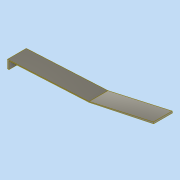
# Autodesk Inventor part: limitSwitchTrigger
Saved by Autodesk Inventor 2017 (Build 210142000, 142)
## iProperties
Created: 2016-12-03
Part Number: limitSwitchTrigger
Material: Steel
Document SubType Name: Modeling
Designer: techn
Density: 7.85 g/cm^3
Appearance: Silver
Author: techn
Autodesk Inventor part; units mm, degrees
ref_plane "YZ Plane" through (0, 0, 0) normal (1, 0, 0) x (0, 1, 0)
ref_plane "XZ Plane" through (0, 0, 0) normal (0, 1, 0) x (-1, 0, 0)
ref_plane "XY Plane" through (0, 0, 0) normal (0, 0, 1) x (1, 0, 0)
sketch "Sketch1" plane through (0, 0, 0) normal (0, 0, 1) x (1, 0, 0)
  line L0 (0, 0) -> (0, 1.016)
  line L1 (0, 1.016) -> (10.8309, 1.5836)
  line L2 (10.8309, 1.5836) -> (19.5267, 3.432)
  line L3 (10.8309, 1.5836) -> (19.7209, 1.5836) construction
  line L4 (19.5267, 3.432) -> (19.4844, 3.6307)
  line L5 (19.4844, 3.6307) -> (10.8098, 1.683)
  line L6 (10.8098, 1.683) -> (0, 1.1162)
  line L7 (0, 1.1162) -> (-0.2029, 1.1056)
  line L8 (-0.2029, 1.1056) -> (-0.2029, 0)
  line L9 (-0.2029, 0) -> (0, 0)
  dimension "d0" = 1.016
  dimension "d1" = 10.8458
  dimension "d2" = 93
  dimension "d3" = 8.89
  dimension "d4" = 12
  dimension "d5" = 0.2032
  dimension "d6" = 0.2032
  constraints: 20 end point, 2 vertical, 1 equal length, 1 horizontal, 1 perpendicular, 1 point on line
  measures "d0" distance of L0.start L0.end
  measures "d1" distance of L0.end L1.end
  measures "d2" angle of L0 L1
  measures "d3" distance of L1.end L2.end
  measures "d4" angle of L3 L2
  measures "d5" distance of L2.end L4.end
  measures "d6" distance of L6.end L7.end
extrude "Extrusion1" add sketch "Sketch1" along normal blind 2.54
body "Solid1"
